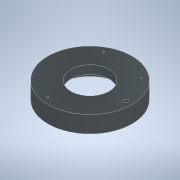
# Autodesk Inventor part: Корпус сальника 4
Saved by Autodesk Inventor 2021 (Build 250183000, 183)
## iProperties
Created: 2020-11-05
Part Number: Корпус сальника 4
Material: Чугун, серый
Document SubType Name: Modeling
Designer: Тимоха
Density: 7.15 g/cm^3
Appearance: Чугун серый
Mass: 1505.16 g
Surface Area: 407.904 cm^2
Volume: 210.512 cm^3
Author: Тимоха
Autodesk Inventor part; units mm, degrees
ref_plane "YZ Plane" through (0, 0, 0) normal (1, 0, 0) x (0, 1, 0)
ref_plane "XZ Plane" through (0, 0, 0) normal (0, 1, 0) x (-1, 0, 0)
ref_plane "XY Plane" through (0, 0, 0) normal (0, 0, 1) x (1, 0, 0)
sketch "Эскиз1" plane through (0, 0, 0) normal (0, 0, 1) x (1, 0, 0)
  line L0 (0, 0) -> (0, 20)
  line L1 (0, 0) -> (0, 24)
  line L2 (0, 0) -> (0, 30)
  line L3 (0, 30) -> (-75, 30)
  line L4 (-75, 30) -> (-75, 0)
  line L5 (-75, 0) -> (-51, 0)
  line L6 (-51, 0) -> (-51, 15)
  line L7 (-51, 15) -> (-34, 15)
  line L8 (-34, 15) -> (-34, 30)
  line L9 (-54, 27) -> (-39, 27)
  line L10 (-39, 27) -> (-39, 20)
  line L11 (-39, 20) -> (-54, 20)
  line L12 (-54, 20) -> (-54, 27)
  dimension "d20" = 30
  dimension "d21" = 75
  dimension "d22" = 24
  dimension "d23" = 15
  dimension "d24" = 17
  dimension "d46" = 7
  dimension "d47" = 3
  constraints: 26 end point, 6 perpendicular, 3 point on line, 2 horizontal, 2 parallel, 1 vertical
  measures "d20" distance of L0.start L2.end
  measures "d21" distance of L2.end L3.end
  measures "d22" distance of L4.end L5.end
  measures "d23" distance of L5.end L6.end
  measures "d24" distance of L6.end L7.end
  measures "d46" distance of L9.end L10.end
  measures "d47" distance between parallel lines of L3 L9
revolve "Вращение1" add sketch "Эскиз1" angle 360 about axis through (0, 0, 0) along (0, 1, 0)
sketch "Эскиз2" plane through (0, 30, 0) normal (0, 1, 0) x (1, 0, 0)
  circle A0 centre (0, 0) radius 32
  circle A1 centre (0, 0) radius 69
  line L0 (0, 0) -> (41.781195, 49.792889)
  line L1 (0, 0) -> (65, 0) construction
  circle A2 centre (41.781195, 49.792889) radius 1.5
  line L2 (0, 0) -> (-32.5, 56.291651)
  line L3 (0, 0) -> (65, 0) construction
  circle A3 centre (-32.5, 56.291651) radius 1.5
  line L4 (0, 0) -> (-11.287132, -64.012504)
  line L5 (0, 0) -> (65, 0) construction
  circle A4 centre (-11.287132, -64.012504) radius 1.5
  dimension "d8" = 65
  dimension "d9" = 50
  dimension "d10" = 3
  dimension "d11" = 65
  dimension "d12" = 120
  dimension "d13" = 3
  dimension "d14" = 65
  dimension "d15" = 100
  dimension "d16" = 3
  constraints: 12 end point, 3 centre point, 3 coincident, 3 equal length, 3 horizontal, 1 point on line
  measures "d8" distance of L0.start L0.end
  measures "d9" angle of L1 L0
  measures "d10" diameter of A2
  measures "d11" distance of L0.start L2.end
  measures "d12" angle of L3 L2
  measures "d13" diameter of A3
  measures "d14" distance of L0.start L4.end
  measures "d15" angle of L4 L5
  measures "d16" diameter of A4
extrude "Выдавливание1" cut sketch "Эскиз2" against normal through all contours A2 | A3 | A4
sketch "Эскиз3" plane through (0, 0, 0) normal (0, 1, 0) x (-1, 0, 0)
  circle A0 centre (11.287132, 64.012504) radius 1.5
  circle A1 centre (-41.781195, -49.792889) radius 1.5
  circle A2 centre (32.5, -56.291651) radius 1.5
  circle A3 centre (0, 0) radius 75
  circle A4 centre (0, 0) radius 34
  circle A5 centre (-64, 0) radius 4
  dimension "d44" = 64
  dimension "d45" = 8
  constraints: 1 centre point
  measures "d44" distance of A5.centre point (0, 0)
  measures "d45" diameter of A5
extrude "Выдавливание2" cut sketch "Эскиз3" along normal through all contours A5
sketch "Эскиз4" plane through (0, 0, 0) normal (0, 1, 0) x (-1, 0, 0)
  circle A0 centre (-64, 0) radius 4 projected
  circle A1 centre (-64, 0) radius 5
  point P0 (0, 0)
  dimension "d27" = 10
  constraints: 1 centre point, 1 coincident
  measures "d27" diameter of A1
extrude "Выдавливание3" cut sketch "Эскиз4" along normal blind 1
sketch "Эскиз5" plane through (0, 0, 0) normal (0, 1, 0) x (-1, 0, 0)
  line L0 (0, 0) -> (64, 0)
  dimension "d30" = 64
  constraints: 2 end point, 1 horizontal
  measures "d30" distance of L0.start L0.end
hole "Отверстие1" at (-64, 0, 0) direction (0, 1, 0) diameter 7.9 depth 23 tip angle 118 counterbore diameter 8 counterbore depth 22
pattern_circular "Круговой массив1" count 2 over 360 about axis through (0, 7.5, 0) along (0, -1, 0) of "Выдавливание3"
sketch "Эскиз6" plane through (0, 0, 0) normal (0, 0, 1) x (1, 0, 0)
  line L0 (-54, 20) -> (54, 20)
  line L1 (-54, 20) -> (-54, 27)
  line L2 (-54, 20) -> (-54, 27)
  line L3 (-60, 1) -> (-60, 22)
  line L4 (-54, 20) -> (-54, 27)
  line L5 (-60, 1) -> (-60, 22)
  line L6 (-54, 20) -> (-60, 20)
  line L7 (-60, 1) -> (-60, 22)
  line L8 (-60, 20) -> (-60, 21.5)
  line L9 (-60, 1) -> (-60, 22)
  line L10 (-60, 21.5) -> (-54, 23.5)
  line L11 (-54, 20) -> (-54, 27)
  line L12 (-54, 23.5) -> (-54, 20.5)
  line L13 (-54, 20) -> (-54, 27)
  line L14 (-54, 20.5) -> (-77.76732, 12.57756)
  line L15 (-77.76732, 12.57756) -> (-78.66732, 15.27756)
  line L16 (-78.66732, 15.27756) -> (-52.512187, 23.995938)
  line L17 (-52.512187, 23.995938) -> (-51.612187, 21.295938)
  line L18 (-51.612187, 21.295938) -> (-54, 20.5)
  point P0 (0, 0)
  dimension "d68" = 1.5
  dimension "d69" = 3
  constraints: 18 end point, 4 perpendicular, 4 point on line, 1 parallel, 6 other
  measures "d68" distance of L6.end L8.end
  measures "d69" distance of L10.end L12.end
revolve "Вращение2" cut sketch "Эскиз6" angle 360 about axis through (-78.66732, 15.27756, 0) along (0.9486833, 0.3162278, 0) contours L14 L6 L3 L10 L1 | L1 L16 L17 L18 | L14 L3 L6 | L3 L14 L15 L16
sketch "Эскиз7" plane through (0, 0, 0) normal (0, 0, 1) x (1, 0, 0)
  line L0 (-34, 15) -> (34, 15) projected
  point P0 (0, 0)
  point P1 (0, 17.5)
  dimension "d55" = 2.5
  measures "d55" distance from line of point (0, 17.5) L0
hole "Отверстие2" at (0, 17.5, 0) direction (0, 0, 1) diameter 3.4 depth 69 tip angle 118 counterbore diameter 3.5 counterbore depth 68.75
sketch "Эскиз8" plane through (0, 0, 0) normal (0, -1, 0) x (1, 0, 0)
  circle A0 centre (0, 0) radius 34 projected
  line L0 (0, 34) -> (0, 67)
  dimension "d56" = 33
  constraints: 2 end point, 1 vertical, 1 vertical alignment, 1 other
  measures "d56" distance of L0.start L0.end
hole "Отверстие3" at (0, 0, 67) direction (0, 1, 0) diameter 3.4 depth 18 tip angle 118 counterbore diameter 4 counterbore depth 17
sketch "Эскиз9" plane through (0, 0, 0) normal (0, -1, 0) x (1, 0, 0)
  circle A0 centre (0, 0) radius 53
  circle A1 centre (0, 0) radius 55
  dimension "d64" = 106
  dimension "d65" = 110
  constraints: 2 centre point, 2 coincident
  measures "d64" diameter of A0
  measures "d65" diameter of A1
extrude "Выдавливание4" cut sketch "Эскиз9" against normal blind 1.5
